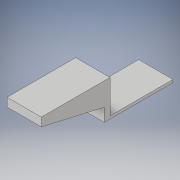
# Autodesk Inventor part: Pillow Holder
Saved by Autodesk Inventor 2017 (Build 210142000, 142)
## iProperties
Created: 2017-01-27
Part Number: Pillow Holder
Material: Generic
Document SubType Name: Modeling
Designer: jbui8
Density: 1 g/cm^3
Appearance: Default
Author: jbui8
Autodesk Inventor part; units mm, degrees
ref_plane "YZ Plane" through (0, 0, 0) normal (1, 0, 0) x (0, 1, 0)
ref_plane "XZ Plane" through (0, 0, 0) normal (0, 1, 0) x (-1, 0, 0)
ref_plane "XY Plane" through (0, 0, 0) normal (0, 0, 1) x (1, 0, 0)
sketch "Sketch1" plane through (0, 0, 0) normal (0, 1, 0) x (-1, 0, 0)
  line L0 (0, 0) -> (76.2, 0)
  line L1 (76.2, 0) -> (76.2, -152.4)
  line L2 (76.2, -152.4) -> (0, -152.4)
  line L3 (0, -152.4) -> (0, 0)
  dimension "d0" = 76.2
  dimension "d1" = 152.4
  constraints: 8 end point, 2 parallel, 1 horizontal, 1 perpendicular
  measures "d0" distance of L1.end L2.end
  measures "d1" distance of L0.end L1.end
extrude "Extrusion1" add sketch "Sketch1" along normal blind 6.35
sketch "Sketch2" plane through (0, 6.35, 0) normal (0, 1, 0) x (1, 0, 0)
  line L0 (-76.2, 152.4) -> (-76.2, 0) projected
  line L1 (0, 0) -> (-76.2, 0)
  line L2 (-76.2, 0) -> (-76.2, 12.7)
  line L3 (-76.2, 12.7) -> (0, 12.7)
  line L4 (0, 12.7) -> (0, 0)
  dimension "d4" = 12.7
  constraints: 8 end point, 2 parallel, 1 horizontal, 1 perpendicular, 1 point on line
  measures "d4" distance of L1.end L2.end
extrude "Extrusion2" add sketch "Sketch2" along normal blind 22.86
sketch "Sketch3" plane through (0, 29.21, 0) normal (0, 1, 0) x (1, 0, 0)
  line L0 (0, 152.4) -> (0, 0) projected
  line L1 (0, 12.7) -> (-76.2, 12.7)
  line L2 (-76.2, 12.7) -> (-76.2, -139.7)
  line L3 (-76.2, -139.7) -> (0, -139.7)
  line L4 (0, -139.7) -> (0, 12.7)
  line L5 (0, 12.7) -> (-76.2, 12.7) projected
  dimension "d7" = 76.2
  dimension "d8" = 152.4
  constraints: 8 end point, 2 parallel, 1 collinear, 1 horizontal, 1 perpendicular, 1 point on line
  measures "d7" distance of L3.end L2.end
  measures "d8" distance of L2.end L1.end
extrude "Extrusion3" add sketch "Sketch3" along normal blind 50.8
sketch "Sketch4" plane through (-76.2, 0, -152.4) normal (-1, 0, 0) x (0, 0, 1)
  line L0 (292.1, 29.21) -> (152.4, 29.21) projected
  line L1 (152.4, 29.21) -> (292.1, 61.1529)
  line L2 (152.4, 0) -> (152.4, 29.21) projected
  line L3 (152.4, 29.21) -> (292.1, 29.21)
  line L4 (292.1, 29.21) -> (292.1, 80.01) projected
  constraints: 4 end point, 2 point on line, 1 perpendicular
extrude "Extrusion4" cut sketch "Sketch4" against normal through all
body "Solid1"
